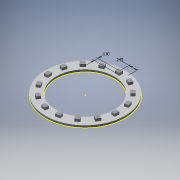
# Autodesk Inventor part: LEDRing
Saved by Autodesk Inventor 2017 (Build 210142000, 142)
## iProperties
Created: 2016-12-05
Part Number: LEDRing
Material: Generic
Document SubType Name: Modeling
Designer: PLTW
Density: 1 g/cm^3
Appearance: Default
Author: PLTW
Autodesk Inventor part; units mm, degrees
ref_plane "YZ Plane" through (0, 0, 0) normal (1, 0, 0) x (0, 1, 0)
ref_plane "XZ Plane" through (0, 0, 0) normal (0, 1, 0) x (-1, 0, 0)
ref_plane "XY Plane" through (0, 0, 0) normal (0, 0, 1) x (1, 0, 0)
sketch "Sketch1" plane through (0, 0, 0) normal (0, 1, 0) x (-1, 0, 0)
  circle A0 centre (0, 0) radius 21.9075
  circle A1 centre (0, 0) radius 29.972
  dimension "d0" = 59.944
  dimension "d1" = 43.815
  constraints: 2 centre point, 2 coincident
  measures "d0" diameter of A1
  measures "d1" diameter of A0
extrude "Extrusion1" add sketch "Sketch1" along normal blind 1.524
sketch "Sketch2" plane through (0, 1.524, 0) normal (0, 1, 0) x (1, 0, 0)
  circle A0 centre (0, 0) radius 21.9075 projected
  line L0 (-1.651, 24.1935) -> (1.651, 24.1935)
  line L1 (1.651, 24.1935) -> (1.651, 26.9935)
  line L2 (1.651, 26.9935) -> (-1.651, 26.9935)
  line L3 (-1.651, 26.9935) -> (-1.651, 24.1935)
  line L4 (-1.651, 24.1935) -> (1.651, 26.9935) construction
  line L5 (1.651, 24.1935) -> (-1.651, 26.9935) construction
  circle A1 centre (0, 0) radius 29.972 projected
  point P0 (0, 25.5935)
  point P1 (0, 25.5935)
  dimension "d4" = 3.302
  dimension "d5" = 2.8
  dimension "d12" = 24.1935
  constraints: 12 end point, 3 midpoint, 2 parallel, 1 horizontal, 1 perpendicular, 1 vertical alignment
  measures "d4" distance of L1.end L2.end
  measures "d5" distance of L0.end L1.end
  measures "d12" distance from line of A1.centre L0
extrude "Extrusion2" add sketch "Sketch2" along normal blind 1.9 contours L3 L2 L1 L0
pattern_circular "Circular Pattern1" count 15 over 360 about axis through (0, 0, 0) along (0, 1, 0) of "Extrusion2"
sketch "Sketch4" plane through (0, 0, 0) normal (1, 0, 0) x (0, 1, 0)
  line L0 (0, -27.432) -> (-0.3048, -27.432)
  line L1 (-0.3048, -27.432) -> (-0.3048, -24.257)
  line L2 (-0.3048, -24.257) -> (0, -24.257)
  line L3 (0, -24.257) -> (0, -27.432)
  line L4 (0, 29.972) -> (0, -29.972) projected
  line L5 (-1.0506, 0) -> (4.1698, 0) projected
  point P0 (0, 0)
  dimension "d21" = 3.175
  dimension "d22" = 0.3048
  dimension "d23" = 2.54
  constraints: 8 end point, 2 parallel, 1 horizontal, 1 perpendicular, 1 point on line
  measures "d21" distance of L0.end L1.end
  measures "d22" distance of L1.end L2.end
  measures "d23" distance from line of L4.end L0
revolve "Revolution1" add sketch "Sketch4" angle 360 about axis through (0, -10, 0) along (0, 1, 0)
ref_plane "Work Plane1" through (-24.2026, 3.424, 12.0669) normal (-0.5, 0, -0.866) x (-0.866, 0, 0.5)
sketch "Sketch5" plane through (-24.2026, 3.424, 12.0669) normal (-0.5, 0, -0.866) x (-0.866, 0, 0.5)
  line L0 (-56.9655, -3.424) -> (2.9785, -3.424) projected
  line L1 (0.4385, -3.424) -> (-54.4255, -3.424) projected
  line L2 (2.6047, -3.424) -> (-4.6343, -3.424)
  line L3 (-4.6343, -3.424) -> (-4.6343, -4.694)
  line L4 (-4.6343, -4.694) -> (2.6047, -4.694)
  line L5 (2.6047, -4.694) -> (2.6047, -3.424)
  line L6 (-26.9935, -5.6328) -> (-26.9935, 0.9388) projected
  point P0 (-26.9935, -3.424)
  dimension "d25" = 1.27
  dimension "d26" = 0.3738
  dimension "d27" = 7.239
  constraints: 8 end point, 2 parallel, 1 horizontal, 1 perpendicular, 1 point on line
  measures "d25" distance of L2.end L3.end
  measures "d26" distance of L0.end L2.start
  measures "d27" distance of L3.end L4.end
revolve "Revolution2" add sketch "Sketch5" angle 5 mid plane about axis through (-0.8255, -10, -1.4298) along (0, 1, 0)
body "Solid1"
